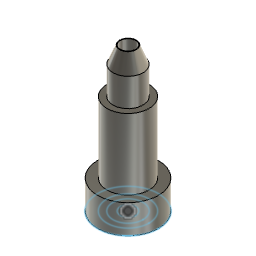
pipette-upper-spring-stopper (Autodesk Fusion 360 design; units mm, degrees)
Autodesk Fusion 360 part; units mm, degrees
sketch "Sketch1" plane through (0, 0, 0) normal (0, 0, 1) x (1, 0, 0)
  circle A0 centre (0, 0) radius 2.25
  circle A1 centre (0, 0) radius 3.15
  circle A2 centre (0, 0) radius 4.55
  circle A3 centre (0, 0) radius 1.15
  dimension "d1" = 9.1
  dimension "d2" = 6.3
  dimension "d3" = 4.5
  dimension "d4" = 2.3
  constraint coincident A0.centre A1.centre
  constraint concentric A1 A2
  constraint concentric A1 A3
  measures "d1" diameter of A2
  measures "d2" diameter of A1
  measures "d3" diameter of A0
  measures "d4" diameter of A3
extrude "Extrude1" add sketch "Sketch1" along normal blind 4.3 contours A0 | A1 | A2 | A3
extrude "Extrude2" add sketch "Sketch1" along normal blind 14.9 contours A0 | A1 | A3
extrude "Extrude3" add sketch "Sketch1" along normal blind 21.6 contours A0 | A3
extrude "Extrude4" cut sketch "Sketch1" along normal up to surface (17.3 mm away) from surface at 4.3 contours A3
chamfer "Chamfer1" distance 1 distance2 2.5 1 edges at (-2.0977, -0.8136, 21.6) measured on face at (1.875, -0.1118, 21.6)
